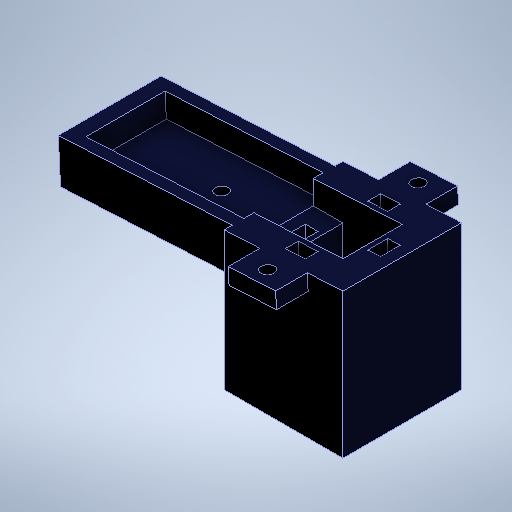
# Autodesk Inventor part: Upper Path Fixation
Saved by Autodesk Inventor 2025.4 (Build 294407000, 407)
## iProperties
Created: 2026-04-10
Part Number: Upper Path Fixation
Material: Generic
Document SubType Name: Modeling
Designer: lenovo
Density: 1 g/cm^3
Appearance: Default(1)
Author: lenovo
Autodesk Inventor part; units mm, degrees
ref_plane "YZ Plane" through (0, 0, 0) normal (1, 0, 0) x (0, 1, 0)
ref_plane "XZ Plane" through (0, 0, 0) normal (0, 1, 0) x (-1, 0, 0)
ref_plane "XY Plane" through (0, 0, 0) normal (0, 0, 1) x (1, 0, 0)
sketch "Sketch1" plane through (0, 0, 0) normal (0, 0, 1) x (1, 0, 0)
  line L0 (-15, -17.5) -> (15, -17.5)
  line L1 (15, -17.5) -> (15, 17.5)
  line L2 (15, 17.5) -> (-15, 17.5)
  line L3 (-15, 17.5) -> (-15, -17.5)
  line L4 (-15, -17.5) -> (15, 17.5) construction
  line L5 (15, -17.5) -> (-15, 17.5) construction
  line L6 (-15, 17.5) -> (15, 19.0722)
  line L7 (15, 19.0722) -> (15, 17.5)
  point P0 (0, 0)
  dimension "d0" = 3
  dimension "d1" = 30
  dimension "d3" = 35
  constraints: 16 end point, 2 midpoint, 2 parallel, 1 horizontal, 1 perpendicular, 1 vertical
  measures "d0" angle of L6 L2
  measures "d1" distance of L0.start L0.end
  measures "d3" distance of L0.end L1.end
extrude "Extrusion1" add sketch "Sketch1" along normal mid plane 30
sketch "Sketch2" plane through (-15, -17.5, -15) normal (0, -1, 0) x (1, 0, 0)
  line L0 (7.5, 7.5) -> (22.5, 7.5)
  line L1 (22.5, 7.5) -> (22.5, 22.5)
  line L2 (22.5, 22.5) -> (7.5, 22.5)
  line L3 (7.5, 22.5) -> (7.5, 7.5)
  line L4 (7.5, 7.5) -> (22.5, 22.5) construction
  line L5 (22.5, 7.5) -> (7.5, 22.5) construction
  line L6 (0, 30) -> (0, 0) projected
  line L7 (30, 0) -> (0, 0) projected
  line L8 (12.5, 3) -> (17.5, 3)
  line L9 (17.5, 3) -> (17.5, 6.2)
  line L10 (17.5, 6.2) -> (12.5, 6.2)
  line L11 (12.5, 6.2) -> (12.5, 3)
  line L12 (12.5, 3) -> (17.5, 6.2) construction
  line L13 (17.5, 3) -> (12.5, 6.2) construction
  line L14 (3, 17.5) -> (6.2, 17.5)
  line L15 (6.2, 17.5) -> (6.2, 12.5)
  line L16 (6.2, 12.5) -> (3, 12.5)
  line L17 (3, 12.5) -> (3, 17.5)
  line L18 (3, 17.5) -> (6.2, 12.5) construction
  line L19 (6.2, 17.5) -> (3, 12.5) construction
  line L20 (15, 7.5) -> (15, 22.5)
  line L21 (7.5, 15) -> (22.5, 15)
  line L22 (12.5, 27) -> (17.5, 27)
  line L23 (17.5, 27) -> (17.5, 23.8)
  line L24 (17.5, 23.8) -> (12.5, 23.8)
  line L25 (12.5, 23.8) -> (12.5, 27)
  line L26 (12.5, 27) -> (17.5, 23.8) construction
  line L27 (17.5, 27) -> (12.5, 23.8) construction
  line L28 (27, 17.5) -> (23.8, 17.5)
  line L29 (23.8, 17.5) -> (23.8, 12.5)
  line L30 (23.8, 12.5) -> (27, 12.5)
  line L31 (27, 12.5) -> (27, 17.5)
  line L32 (27, 17.5) -> (23.8, 12.5) construction
  line L33 (23.8, 17.5) -> (27, 12.5) construction
  point P0 (15, 15)
  point P1 (15, 15)
  point P2 (0, 15)
  point P3 (15, 0)
  point P4 (15, 4.6)
  point P5 (4.6, 15)
  point P6 (0, 15)
  point P7 (3, 15)
  point P8 (15, 0)
  point P9 (15, 25.4)
  point P10 (25.4, 15)
  point P11 (27, 15)
  dimension "d6" = 15
  dimension "d7" = 5
  dimension "d8" = 3.2
  dimension "d9" = 3
  dimension "d10" = 3
  constraints: 64 end point, 13 midpoint, 11 symmetric about line, 6 parallel, 6 perpendicular, 3 horizontal, 2 horizontal alignment, 2 vertical alignment, 3 other
  measures "d6" distance of L1.end L2.end
  measures "d7" distance of L16.end L14.start
  measures "d8" distance of L14.start L14.end
  measures "d9" distance between parallel lines of L6 L17
  measures "d10" distance of the line from the sketch origin of L8
extrude "Extrusion2" cut sketch "Sketch2" against normal through all
sketch "Sketch3" plane through (0, 0, 0) normal (0, 0, 1) x (1, 0, 0)
  line L0 (-15, -17.5) -> (-15, 17.5) projected
  line L1 (-15, 6.4849) -> (-58.364, 4.2123)
  line L2 (-58.364, 4.2123) -> (-58.9397, 15.1972)
  line L3 (-58.9397, 15.1972) -> (-54.9452, 15.4066)
  line L4 (-54.9452, 15.4066) -> (-54.6312, 9.4148)
  line L5 (-54.6312, 9.4148) -> (-15, 11.4918)
  line L6 (15, 19.0722) -> (-15, 17.5) projected
  line L7 (-54.9452, 15.4066) -> (-15, 17.5)
  point P0 (0, 0)
  dimension "d14" = 4
  dimension "d15" = 5
  dimension "d16" = 6
  dimension "d17" = 40
  constraints: 12 end point, 3 parallel, 2 collinear, 2 point on line, 1 perpendicular
  measures "d14" distance of L2.end L3.end
  measures "d15" distance from line of L1 L5.end
  measures "d16" distance from line of L6 L5.end
  measures "d17" distance of L0.end L3.end
extrude "Extrusion3" add sketch "Sketch3" along normal mid plane 20 contours L1 L2 L3 L4 L5 L0
sketch "Sketch4" plane through (-54.6312, 9.4148, 10) normal (-0.0523, 0.9986, 0) x (0.9986, 0.0523, 0)
  circle A0 centre (24, 10) radius 1.6
  line L0 (39.6856, 20) -> (39.6856, 0) projected
  line L1 (0, 0) -> (0, 20) projected
  point P0 (54.0636, 10)
  point P1 (39.6856, 10)
  dimension "d20" = 3.2
  dimension "d21" = 24
  constraints: 1 centre point, 1 horizontal alignment, 1 midpoint
  measures "d20" diameter of A0
  measures "d21" distance from line of A0.centre L1
extrude "Extrusion4" cut sketch "Sketch4" against normal blind 20
sketch "Sketch5" plane through (-15, -17.5, 15) normal (-1, 0, 0) x (0, 0, 1)
  line L0 (-22.5, 36.9918) -> (-7.5, 36.9918)
  line L1 (-7.5, 36.9918) -> (-7.5, 28.9918)
  line L2 (-7.5, 28.9918) -> (-22.5, 28.9918)
  line L3 (-22.5, 28.9918) -> (-22.5, 36.9918)
  line L4 (-22.5, 36.9918) -> (-7.5, 28.9918) construction
  line L5 (-7.5, 36.9918) -> (-22.5, 28.9918) construction
  line L6 (-30, 35) -> (0, 35) projected
  line L7 (-25, 28.9918) -> (-5, 28.9918) projected
  point P0 (-15, 17.5)
  point P1 (-15, 32.9918)
  point P2 (-15, 35)
  point P3 (-15, 28.9918)
  dimension "d24" = 15
  dimension "d25" = 8
  constraints: 12 end point, 5 midpoint, 2 parallel, 1 horizontal, 1 perpendicular, 1 vertical alignment
  measures "d24" distance of L0.start L0.end
  measures "d25" distance of L0.end L1.end
extrude "Extrusion5" cut sketch "Sketch5" against normal up to surface (22.5 mm away)
sketch "Sketch7" plane through (0, 0, 15) normal (0, 0, 1) x (1, 0, 0)
  line L0 (15, 19.0722) -> (-15, 17.5) projected
  line L1 (-5.9918, 17.9721) -> (5.9918, 18.6001)
  line L2 (5.9918, 18.6001) -> (6.2011, 14.6056)
  line L3 (6.2011, 14.6056) -> (-5.7824, 13.9776)
  line L4 (-5.7824, 13.9776) -> (-5.9918, 17.9721)
  line L5 (-5.9918, 17.9721) -> (6.2011, 14.6056) construction
  line L6 (5.9918, 18.6001) -> (-5.7824, 13.9776) construction
  point P0 (0, 0)
  point P1 (0, 18.2861)
  point P2 (0.1047, 16.2889)
  point P3 (0, 18.2861)
  point P4 (5.9918, 18.6001)
  point P5 (-5.9918, 17.9721)
  dimension "d30" = 12
  dimension "d31" = 4
  constraints: 12 end point, 5 midpoint, 2 parallel, 1 collinear, 1 perpendicular
  measures "d30" distance of L2.end L3.end
  measures "d31" distance of L1.end L2.end
extrude "Extrusion6" add sketch "Sketch7" along normal blind 8
sketch "Sketch8" plane through (15, 19.0722, 15) normal (-0.0523, 0.9986, 0) x (0.9986, 0.0523, 0)
  circle A0 centre (-15.0206, -4) radius 1.65
  line L0 (-9.0206, 0) -> (-9.0206, -8) projected
  line L1 (-9.0206, -8) -> (-21.0206, -8) projected
  line L2 (-9.0206, 0) -> (-21.0206, 0) projected
  point P0 (-15.9776, 15)
  point P1 (-9.0206, -4)
  point P2 (-15.0206, -8)
  point P3 (-15.0206, 0)
  dimension "d34" = 3.3
  dimension "d37" = 4
  constraints: 3 midpoint, 1 centre point, 1 vertical alignment
  measures "d34" diameter of A0
  measures "d37" distance of point (-15.021, 0) A0.centre
extrude "Extrusion7" cut sketch "Sketch8" against normal blind 12
mirror "Mirror1" about plane through (0, 0, 0) normal (0, 0, 1) of "Extrusion6", "Extrusion7"
extrude "Extrusion8" add sketch "Sketch3" along normal blind 3 from surface at 10
mirror "Mirror2" about plane through (0, 0, 0) normal (0, 0, 1) of "Extrusion8"
equation "\"d10\" = d9"
body "Solid1"
